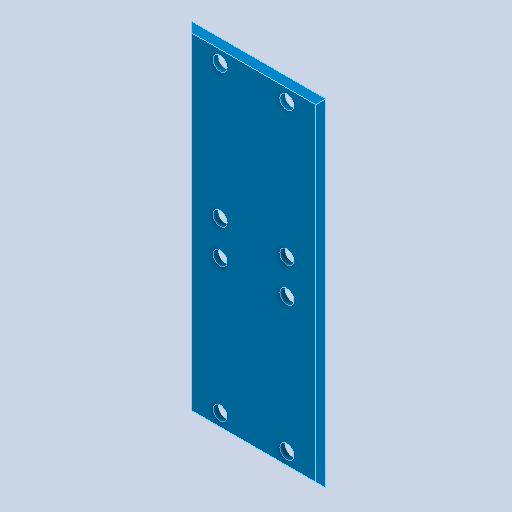
# Autodesk Inventor part: Panel Side 1x2
Saved by Autodesk Inventor 2023.1 (Build 271208000, 208)
## iProperties
Created: 2022-08-10
Part Number: Panel Side 1x2
Material: Generic
Document SubType Name: Modeling
Designer: xSibe
Density: 1 g/cm^3
Appearance: Plastic Teal
Author: xSibe
Autodesk Inventor part; units mm, degrees
ref_plane "YZ Plane" through (0, 0, 0) normal (1, 0, 0) x (0, 1, 0)
ref_plane "XZ Plane" through (0, 0, 0) normal (0, 1, 0) x (-1, 0, 0)
sketch "Sketch1" plane through (0, 0, 0) normal (0, 0, 1) x (1, 0, 0)
  line L0 (49.8, -22.9) -> (49.8, 22.9) projected
  line L1 (42.1, 24.9) -> (0.75, 24.9) projected
  line L2 (0.75, -24.9) -> (42.1, -24.9) projected
  line L3 (0, 22.9) -> (0, -22.9) projected
  line L4 (0.75, -22.9) -> (0.75, 22.9) projected
  line L5 (42.1, -22.9) -> (0.75, -22.9) projected
  line L6 (42.1, -22.9) -> (42.1, -17.05) projected
  line L7 (7.7, -17.05) -> (42.1, -17.05) projected
  line L8 (7.7, 17.05) -> (7.7, -17.05) projected
  line L9 (7.7, 17.05) -> (42.1, 17.05) projected
  line L10 (42.1, 17.05) -> (42.1, 22.9) projected
  line L11 (0.75, 22.9) -> (42.1, 22.9) projected
  circle A0 centre (34.8, -19.9) radius 2.0625 projected
  circle A1 centre (34.8, 19.9) radius 2.0625 projected
  circle A2 centre (15, -19.9) radius 2.0625 projected
  circle A3 centre (15, 19.9) radius 2.0625 projected
  line L12 (24.9, 17.05) -> (24.9, -17.05)
  line L13 (4.9, 25) -> (44.9, 25)
  line L14 (44.9, 25) -> (44.9, -25)
  line L15 (44.9, -25) -> (4.9, -25)
  line L16 (4.9, -25) -> (4.9, 25)
  line L17 (4.9, 25) -> (44.9, -25) construction
  line L18 (44.9, 25) -> (4.9, -25) construction
  point P0 (0, 0)
  point P1 (24.9, 0)
  dimension "d0" = 40
  dimension "d1" = 50
  constraints: 14 end point, 5 midpoint, 2 parallel, 1 horizontal, 1 perpendicular
  measures "d0" distance of L14.end L15.end
  measures "d1" distance of L13.end L14.end
ref_plane "Work Plane1" through (0.75, -22.9, 24.9) normal (0, 0, 1) x (1, 0, 0)
extrude "Extrusion1" add sketch "Sketch1" along normal blind 1.5 from surface at 24.9 contours L16 L11 L10 L9 L8 L7 L6 L5 | L5 L6 L7 L12 L9 L10 L11 L16 L13 L14 L15 | L7 L8 L9 L12
pattern_linear "Rectangular Pattern1" count 2 spacing 50 along (0, 1, 0) of "Extrusion1"
chamfer "Chamfer1" distance 1.5 angle 45 4 edges at (24.9, -25, 26.4) (44.9, 25, 26.4) (4.9, 25, 26.4) (24.9, 75, 26.4)
body "Solid1"
